Autodesk Inventor part; units mm, degrees
(part 9 of 11)
  line L1735 (12.5917, 6.0093) -> (11.97, 5.7878)
  arc A3472 (11.9573, 5.8237) -> (11.9828, 5.7519) centre (11.97, 5.7878) ccw
  arc A3473 (12.6045, 5.9734) -> (12.579, 6.0452) centre (12.5917, 6.0093) ccw
  line L1736 (11.97, 5.7878) -> (11.3254, 5.6466)
  arc A3474 (11.3172, 5.6838) -> (11.3335, 5.6094) centre (11.3254, 5.6466) ccw
  arc A3475 (11.9782, 5.7506) -> (11.9619, 5.825) centre (11.97, 5.7878) ccw
  line L1737 (11.3254, 5.6466) -> (10.668, 5.588)
  arc A3476 (10.6646, 5.626) -> (10.6714, 5.5501) centre (10.668, 5.588) ccw
  arc A3477 (11.3288, 5.6087) -> (11.322, 5.6846) centre (11.3254, 5.6466) ccw
  line L1738 (10.668, 5.588) -> (10.668, 6.858)
  arc A3478 (10.7061, 6.858) -> (10.6299, 6.858) centre (10.668, 6.858) ccw
  arc A3479 (10.6299, 5.588) -> (10.7061, 5.588) centre (10.668, 5.588) ccw
  line L1739 (10.668, 6.858) -> (11.1934, 6.8774)
  arc A3480 (11.1948, 6.8393) -> (11.192, 6.9155) centre (11.1934, 6.8774) ccw
  arc A3481 (10.6666, 6.8961) -> (10.6694, 6.8199) centre (10.668, 6.858) ccw
  line L1740 (11.1934, 6.8774) -> (11.7108, 6.9714)
  arc A3482 (11.7176, 6.9339) -> (11.704, 7.0089) centre (11.7108, 6.9714) ccw
  arc A3483 (11.1866, 6.9149) -> (11.2003, 6.8399) centre (11.1934, 6.8774) ccw
  line L1741 (11.7108, 6.9714) -> (12.2094, 7.1381)
  arc A3484 (12.2215, 7.1019) -> (12.1974, 7.1742) centre (12.2094, 7.1381) ccw
  arc A3485 (11.6987, 7.0075) -> (11.7228, 6.9353) centre (11.7108, 6.9714) ccw
  line L1742 (12.2094, 7.1381) -> (12.6793, 7.374)
  arc A3486 (12.6964, 7.34) -> (12.6623, 7.4081) centre (12.6794, 7.374) ccw
  arc A3487 (12.1924, 7.1721) -> (12.2265, 7.104) centre (12.2094, 7.1381) ccw
  line L1743 (12.6793, 7.374) -> (13.1109, 7.6744)
  arc A3488 (13.1326, 7.6431) -> (13.0891, 7.7057) centre (13.1109, 7.6744) ccw
  arc A3489 (12.6576, 7.4053) -> (12.7011, 7.3427) centre (12.6793, 7.374) ccw
  line L1744 (13.1109, 7.6744) -> (13.4952, 8.0332)
  arc A3490 (13.5212, 8.0053) -> (13.4693, 8.061) centre (13.4952, 8.0332) ccw
  arc A3491 (13.0849, 7.7023) -> (13.1369, 7.6465) centre (13.1109, 7.6744) ccw
  line L1745 (13.4952, 8.0332) -> (13.8247, 8.443)
  arc A3492 (13.8544, 8.4191) -> (13.795, 8.4669) centre (13.8247, 8.443) ccw
  arc A3493 (13.4655, 8.057) -> (13.5249, 8.0093) centre (13.4952, 8.0332) ccw
  line L1746 (13.8247, 8.443) -> (14.0924, 8.8955)
  arc A3494 (14.1252, 8.8761) -> (14.0596, 8.9149) centre (14.0924, 8.8955) ccw
  arc A3495 (13.7919, 8.4624) -> (13.8575, 8.4236) centre (13.8247, 8.443) ccw
  line L1747 (14.0924, 8.8955) -> (14.293, 9.3815)
  arc A3496 (14.3282, 9.367) -> (14.2578, 9.3961) centre (14.293, 9.3815) ccw
  arc A3497 (14.0572, 8.91) -> (14.1276, 8.881) centre (14.0924, 8.8955) ccw
  line L1748 (14.293, 9.3815) -> (14.4224, 9.8911)
  arc A3498 (14.4594, 9.8818) -> (14.3855, 9.9005) centre (14.4224, 9.8911) ccw
  arc A3499 (14.2561, 9.3909) -> (14.33, 9.3721) centre (14.293, 9.3815) ccw
  line L1749 (14.4224, 9.8911) -> (14.478, 10.414)
  arc A3500 (14.5159, 10.41) -> (14.4401, 10.418) centre (14.478, 10.414) ccw
  arc A3501 (14.3845, 9.8952) -> (14.4603, 9.8871) centre (14.4224, 9.8911) ccw
  line L1750 (14.478, 10.414) -> (14.478, 10.668)
  arc A3502 (14.5161, 10.668) -> (14.4399, 10.668) centre (14.478, 10.668) ccw
  arc A3503 (14.4399, 10.414) -> (14.5161, 10.414) centre (14.478, 10.414) ccw
  line L1751 (14.478, 10.668) -> (14.4392, 11.2102)
  arc A3504 (14.4772, 11.2129) -> (14.4012, 11.2075) centre (14.4392, 11.2102) ccw
  arc A3505 (14.44, 10.6653) -> (14.516, 10.6707) centre (14.478, 10.668) ccw
  line L1752 (14.4392, 11.2102) -> (14.3237, 11.7414)
  arc A3506 (14.3609, 11.7495) -> (14.2864, 11.7333) centre (14.3237, 11.7414) ccw
  arc A3507 (14.402, 11.2021) -> (14.4764, 11.2183) centre (14.4392, 11.2102) ccw
  line L1753 (14.3237, 11.7414) -> (14.1337, 12.2507)
  arc A3508 (14.1694, 12.264) -> (14.098, 12.2374) centre (14.1337, 12.2507) ccw
  arc A3509 (14.288, 11.7281) -> (14.3594, 11.7547) centre (14.3237, 11.7414) ccw
  line L1754 (14.1337, 12.2507) -> (13.8732, 12.7278)
  arc A3510 (13.9066, 12.7461) -> (13.8397, 12.7096) centre (13.8732, 12.7278) ccw
  arc A3511 (14.1003, 12.2325) -> (14.1671, 12.269) centre (14.1337, 12.2507) ccw
  line L1755 (13.8732, 12.7278) -> (13.5474, 13.163)
  arc A3512 (13.5779, 13.1859) -> (13.5169, 13.1402) centre (13.5474, 13.163) ccw
  arc A3513 (13.8427, 12.705) -> (13.9037, 12.7507) centre (13.8732, 12.7278) ccw
  line L1756 (13.5474, 13.163) -> (13.163, 13.5474)
  arc A3514 (13.19, 13.5743) -> (13.1361, 13.5205) centre (13.163, 13.5474) ccw
  arc A3515 (13.5205, 13.1361) -> (13.5743, 13.19) centre (13.5474, 13.163) ccw
  line L1757 (13.163, 13.5474) -> (12.7278, 13.8732)
  arc A3516 (12.7507, 13.9037) -> (12.705, 13.8427) centre (12.7278, 13.8732) ccw
  arc A3517 (13.1402, 13.5169) -> (13.1859, 13.5779) centre (13.163, 13.5474) ccw
  line L1758 (12.7278, 13.8732) -> (12.2507, 14.1337)
  arc A3518 (12.269, 14.1671) -> (12.2325, 14.1003) centre (12.2507, 14.1337) ccw
  arc A3519 (12.7096, 13.8397) -> (12.7461, 13.9066) centre (12.7278, 13.8732) ccw
  line L1759 (12.2507, 14.1337) -> (11.7414, 14.3237)
  arc A3520 (11.7547, 14.3594) -> (11.7281, 14.288) centre (11.7414, 14.3237) ccw
  arc A3521 (12.2374, 14.098) -> (12.264, 14.1694) centre (12.2507, 14.1337) ccw
  line L1760 (11.7414, 14.3237) -> (11.2102, 14.4392)
  arc A3522 (11.2183, 14.4764) -> (11.2021, 14.402) centre (11.2102, 14.4392) ccw
  arc A3523 (11.7333, 14.2864) -> (11.7495, 14.3609) centre (11.7414, 14.3237) ccw
  line L1761 (11.2102, 14.4392) -> (10.668, 14.478)
  arc A3524 (10.6707, 14.516) -> (10.6653, 14.44) centre (10.668, 14.478) ccw
  arc A3525 (11.2075, 14.4012) -> (11.2129, 14.4772) centre (11.2102, 14.4392) ccw
  line L1762 (10.668, 14.478) -> (10.1258, 14.4392)
  arc A3526 (10.1231, 14.4772) -> (10.1285, 14.4012) centre (10.1258, 14.4392) ccw
  arc A3527 (10.6707, 14.44) -> (10.6653, 14.516) centre (10.668, 14.478) ccw
  line L1763 (10.1258, 14.4392) -> (9.5946, 14.3237)
  arc A3528 (9.5865, 14.3609) -> (9.6027, 14.2864) centre (9.5946, 14.3237) ccw
  arc A3529 (10.1339, 14.402) -> (10.1177, 14.4764) centre (10.1258, 14.4392) ccw
  line L1764 (9.5946, 14.3237) -> (9.0853, 14.1337)
  arc A3530 (9.072, 14.1694) -> (9.0986, 14.098) centre (9.0853, 14.1337) ccw
  arc A3531 (9.6079, 14.288) -> (9.5813, 14.3593) centre (9.5946, 14.3237) ccw
  line L1765 (9.0853, 14.1337) -> (8.6082, 13.8732)
  arc A3532 (8.5899, 13.9066) -> (8.6264, 13.8397) centre (8.6082, 13.8732) ccw
  arc A3533 (9.1035, 14.1003) -> (9.067, 14.1671) centre (9.0853, 14.1337) ccw
  line L1766 (8.6082, 13.8732) -> (8.173, 13.5474)
  arc A3534 (8.1501, 13.5779) -> (8.1958, 13.5169) centre (8.173, 13.5474) ccw
  arc A3535 (8.631, 13.8427) -> (8.5853, 13.9037) centre (8.6082, 13.8732) ccw
  line L1767 (8.173, 13.5474) -> (7.7886, 13.163)
  arc A3536 (7.7617, 13.19) -> (7.8155, 13.1361) centre (7.7886, 13.163) ccw
  arc A3537 (8.1999, 13.5205) -> (8.146, 13.5743) centre (8.173, 13.5474) ccw
  line L1768 (7.7886, 13.163) -> (7.4628, 12.7278)
  arc A3538 (7.4323, 12.7507) -> (7.4933, 12.705) centre (7.4628, 12.7278) ccw
  arc A3539 (7.8191, 13.1402) -> (7.7581, 13.1859) centre (7.7886, 13.163) ccw
  line L1769 (7.4628, 12.7278) -> (7.2023, 12.2507)
  arc A3540 (7.1689, 12.269) -> (7.2357, 12.2325) centre (7.2023, 12.2507) ccw
  arc A3541 (7.4963, 12.7096) -> (7.4294, 12.7461) centre (7.4628, 12.7278) ccw
  line L1770 (7.2023, 12.2507) -> (7.0123, 11.7414)
  arc A3542 (6.9766, 11.7547) -> (7.048, 11.7281) centre (7.0123, 11.7414) ccw
  arc A3543 (7.238, 12.2374) -> (7.1666, 12.264) centre (7.2023, 12.2507) ccw
  line L1771 (7.0123, 11.7414) -> (6.8968, 11.2102)
  arc A3544 (6.8596, 11.2183) -> (6.934, 11.2021) centre (6.8968, 11.2102) ccw
  arc A3545 (7.0496, 11.7333) -> (6.9751, 11.7495) centre (7.0123, 11.7414) ccw
  line L1772 (6.8968, 11.2102) -> (6.858, 10.668)
  arc A3546 (6.82, 10.6707) -> (6.896, 10.6653) centre (6.858, 10.668) ccw
  arc A3547 (6.9348, 11.2075) -> (6.8588, 11.2129) centre (6.8968, 11.2102) ccw
  line L1773 (6.858, 10.668) -> (6.8782, 10.1815)
  arc A3548 (6.8402, 10.18) -> (6.9163, 10.1831) centre (6.8782, 10.1815) ccw
  arc A3549 (6.8961, 10.6696) -> (6.8199, 10.6664) centre (6.858, 10.668) ccw
  line L1774 (6.8782, 10.1815) -> (6.9618, 9.7019)
  arc A3550 (6.9242, 9.6953) -> (6.9993, 9.7084) centre (6.9618, 9.7019) ccw
  arc A3551 (6.9158, 10.1881) -> (6.8407, 10.175) centre (6.8782, 10.1815) ccw
  line L1775 (6.9618, 9.7019) -> (7.1072, 9.2372)
  arc A3552 (7.0709, 9.2258) -> (7.1436, 9.2486) centre (7.1072, 9.2372) ccw
  arc A3553 (6.9982, 9.7133) -> (6.9254, 9.6905) centre (6.9618, 9.7019) ccw
  line L1776 (7.1072, 9.2372) -> (7.3121, 8.7955)
  arc A3554 (7.2775, 8.7795) -> (7.3466, 8.8116) centre (7.3121, 8.7955) ccw
  arc A3555 (7.1418, 9.2533) -> (7.0727, 9.2212) centre (7.1072, 9.2372) ccw
  line L1777 (7.3121, 8.7955) -> (7.5728, 8.3843)
  arc A3556 (7.5407, 8.364) -> (7.605, 8.4047) centre (7.5728, 8.3843) ccw
  arc A3557 (7.3443, 8.8159) -> (7.2799, 8.7751) centre (7.3121, 8.7955) ccw
  line L1778 (7.5728, 8.3843) -> (7.885, 8.0107)
  arc A3558 (7.8558, 7.9863) -> (7.9143, 8.0352) centre (7.885, 8.0107) ccw
  arc A3559 (7.6021, 8.4088) -> (7.5436, 8.3599) centre (7.5728, 8.3843) ccw
  line L1779 (7.885, 8.0107) -> (8.2433, 7.6811)
  arc A3560 (8.2175, 7.653) -> (8.2691, 7.7091) centre (8.2433, 7.6811) ccw
  arc A3561 (7.9108, 8.0388) -> (7.8592, 7.9827) centre (7.885, 8.0107) ccw
  line L1780 (8.2433, 7.6811) -> (8.6416, 7.401)
  arc A3562 (8.6196, 7.3698) -> (8.6635, 7.4321) centre (8.6416, 7.401) ccw
  arc A3563 (8.2652, 7.7122) -> (8.2214, 7.6499) centre (8.2433, 7.6811) ccw
  line L1781 (8.6416, 7.401) -> (9.073, 7.1753)
  arc A3564 (9.0553, 7.1415) -> (9.0906, 7.209) centre (9.073, 7.1753) ccw
  arc A3565 (8.6592, 7.4347) -> (8.6239, 7.3672) centre (8.6416, 7.401) ccw
  line L1782 (9.073, 7.1753) -> (9.27, 7.6205)
  arc A3566 (9.517, 6.972) -> (9.5432, 7.0436) centre (9.5301, 7.0078) ccw
  arc A3567 (9.0861, 7.211) -> (9.0599, 7.1395) centre (9.073, 7.1753) ccw
  line L1783 (9.27, 7.6205) -> (9.4072, 8.0877)
  arc A3568 (9.3988, 8.0505) -> (9.4155, 8.1249) centre (9.4072, 8.0877) ccw
  arc A3569 (9.2783, 7.6577) -> (9.2616, 7.5833) centre (9.27, 7.6205) ccw
  line L1784 (9.4072, 8.0877) -> (10.4902, 6.858)
  arc A3570 (10.4868, 6.8201) -> (10.4936, 6.896) centre (10.4902, 6.858) ccw
  arc A3571 (9.4106, 8.1256) -> (9.4038, 8.0497) centre (9.4072, 8.0877) ccw
  line L1785 (10.4902, 6.858) -> (10.4902, 5.588)
  arc A3572 (10.4521, 5.588) -> (10.5283, 5.588) centre (10.4902, 5.588) ccw
  arc A3573 (10.5283, 6.858) -> (10.4521, 6.858) centre (10.4902, 6.858) ccw
  line L1786 (9.9806, 15.6972) -> (11.3554, 15.6972)
  arc A3574 (11.3554, 15.6591) -> (11.3554, 15.7353) centre (11.3554, 15.6972) ccw
  arc A3575 (9.9806, 15.7353) -> (9.9806, 15.6591) centre (9.9806, 15.6972) ccw
  line L1787 (9.2739, 15.5448) -> (12.0621, 15.5448)
  arc A3576 (12.0621, 15.5067) -> (12.0621, 15.5829) centre (12.0621, 15.5448) ccw
  arc A3577 (9.2739, 15.5829) -> (9.2739, 15.5067) centre (9.2739, 15.5448) ccw
  line L1788 (8.81, 15.3924) -> (12.526, 15.3924)
  arc A3578 (12.526, 15.3543) -> (12.526, 15.4305) centre (12.526, 15.3924) ccw
  arc A3579 (8.81, 15.4305) -> (8.81, 15.3543) centre (8.81, 15.3924) ccw
  line L1789 (8.4714, 15.24) -> (12.8646, 15.24)
  arc A3580 (12.8646, 15.2019) -> (12.8646, 15.2781) centre (12.8646, 15.24) ccw
  arc A3581 (8.4714, 15.2781) -> (8.4714, 15.2019) centre (8.4714, 15.24) ccw
  line L1790 (8.1773, 15.0876) -> (13.1587, 15.0876)
  arc A3582 (13.1587, 15.0495) -> (13.1587, 15.1257) centre (13.1587, 15.0876) ccw
  arc A3583 (8.1773, 15.1257) -> (8.1773, 15.0495) centre (8.1773, 15.0876) ccw
  line L1791 (7.9252, 14.9352) -> (13.4108, 14.9352)
  arc A3584 (13.4108, 14.8971) -> (13.4108, 14.9733) centre (13.4108, 14.9352) ccw
  arc A3585 (7.9252, 14.9733) -> (7.9252, 14.8971) centre (7.9252, 14.9352) ccw
  line L1792 (7.698, 14.7828) -> (13.638, 14.7828)
  arc A3586 (13.638, 14.7447) -> (13.638, 14.8209) centre (13.638, 14.7828) ccw
  arc A3587 (7.698, 14.8209) -> (7.698, 14.7447) centre (7.698, 14.7828) ccw
  line L1793 (7.5035, 14.6304) -> (13.8325, 14.6304)
  arc A3588 (13.8325, 14.5923) -> (13.8325, 14.6685) centre (13.8325, 14.6304) ccw
  arc A3589 (7.5035, 14.6685) -> (7.5035, 14.5923) centre (7.5035, 14.6304) ccw
  line L1794 (7.309, 14.478) -> (10.668, 14.478)
  arc A3590 (10.668, 14.4399) -> (10.668, 14.5161) centre (10.668, 14.478) ccw
  arc A3591 (7.309, 14.5161) -> (7.309, 14.4399) centre (7.309, 14.478) ccw
  line L1795 (10.668, 14.478) -> (14.027, 14.478)
  arc A3592 (14.027, 14.4399) -> (14.027, 14.5161) centre (14.027, 14.478) ccw
  arc A3593 (10.668, 14.5161) -> (10.668, 14.4399) centre (10.668, 14.478) ccw
  line L1796 (7.1545, 14.3256) -> (9.6035, 14.3256)
  arc A3594 (9.6035, 14.2875) -> (9.6035, 14.3637) centre (9.6035, 14.3256) ccw
  arc A3595 (7.1545, 14.3637) -> (7.1545, 14.2875) centre (7.1545, 14.3256) ccw
  line L1797 (11.7325, 14.3256) -> (14.1815, 14.3256)
  arc A3596 (14.1815, 14.2875) -> (14.1815, 14.3637) centre (14.1815, 14.3256) ccw
  arc A3597 (11.7325, 14.3637) -> (11.7325, 14.2875) centre (11.7325, 14.3256) ccw
  line L1798 (7.0021, 14.1732) -> (9.1912, 14.1732)
  arc A3598 (9.1912, 14.1351) -> (9.1912, 14.2113) centre (9.1912, 14.1732) ccw
  arc A3599 (7.0021, 14.2113) -> (7.0021, 14.1351) centre (7.0021, 14.1732) ccw
  line L1799 (12.1448, 14.1732) -> (14.3339, 14.1732)
  arc A3600 (14.3339, 14.1351) -> (14.3339, 14.2113) centre (14.3339, 14.1732) ccw
  arc A3601 (12.1448, 14.2113) -> (12.1448, 14.1351) centre (12.1448, 14.1732) ccw
  line L1800 (6.8532, 14.0208) -> (8.8785, 14.0208)
  arc A3602 (8.8785, 13.9827) -> (8.8785, 14.0589) centre (8.8785, 14.0208) ccw
  arc A3603 (6.8532, 14.0589) -> (6.8532, 13.9827) centre (6.8532, 14.0208) ccw
  line L1801 (12.4575, 14.0208) -> (14.4829, 14.0208)
  arc A3604 (14.4829, 13.9827) -> (14.4829, 14.0589) centre (14.4829, 14.0208) ccw
  arc A3605 (12.4575, 14.0589) -> (12.4575, 13.9827) centre (12.4575, 14.0208) ccw
  line L1802 (6.7337, 13.8684) -> (8.6018, 13.8684)
  arc A3606 (8.6018, 13.8303) -> (8.6018, 13.9065) centre (8.6018, 13.8684) ccw
  arc A3607 (6.7337, 13.9065) -> (6.7337, 13.8303) centre (6.7337, 13.8684) ccw
  line L1803 (12.7342, 13.8684) -> (14.6023, 13.8684)
  arc A3608 (14.6023, 13.8303) -> (14.6023, 13.9065) centre (14.6023, 13.8684) ccw
  arc A3609 (12.7342, 13.9065) -> (12.7342, 13.8303) centre (12.7342, 13.8684) ccw
  line L1804 (6.6143, 13.716) -> (8.3982, 13.716)
  arc A3610 (8.3982, 13.6779) -> (8.3982, 13.7541) centre (8.3982, 13.716) ccw
  arc A3611 (6.6143, 13.7541) -> (6.6143, 13.6779) centre (6.6143, 13.716) ccw
  line L1805 (12.9378, 13.716) -> (14.7217, 13.716)
  arc A3612 (14.7217, 13.6779) -> (14.7217, 13.7541) centre (14.7217, 13.716) ccw
  arc A3613 (12.9378, 13.7541) -> (12.9378, 13.6779) centre (12.9378, 13.716) ccw
  line L1806 (6.4949, 13.5636) -> (8.1946, 13.5636)
  arc A3614 (8.1946, 13.5255) -> (8.1946, 13.6017) centre (8.1946, 13.5636) ccw
  arc A3615 (6.4949, 13.6017) -> (6.4949, 13.5255) centre (6.4949, 13.5636) ccw
  line L1807 (13.1414, 13.5636) -> (14.8411, 13.5636)
  arc A3616 (14.8411, 13.5255) -> (14.8411, 13.6017) centre (14.8411, 13.5636) ccw
  arc A3617 (13.1414, 13.6017) -> (13.1414, 13.5255) centre (13.1414, 13.5636) ccw
  line L1808 (6.4011, 13.4112) -> (8.0368, 13.4112)
  arc A3618 (8.0368, 13.3731) -> (8.0368, 13.4493) centre (8.0368, 13.4112) ccw
  arc A3619 (6.4011, 13.4493) -> (6.4011, 13.3731) centre (6.4011, 13.4112) ccw
  line L1809 (13.2992, 13.4113) -> (14.935, 13.4112)
  arc A3620 (14.935, 13.3731) -> (14.935, 13.4493) centre (14.935, 13.4112) ccw
  arc A3621 (13.2992, 13.4494) -> (13.2992, 13.3732) centre (13.2992, 13.4113) ccw
  line L1810 (6.3089, 13.2588) -> (7.8844, 13.2588)
  arc A3622 (7.8844, 13.2207) -> (7.8844, 13.2969) centre (7.8844, 13.2588) ccw
  arc A3623 (6.3089, 13.2969) -> (6.3089, 13.2207) centre (6.3089, 13.2588) ccw
  line L1811 (13.4516, 13.2589) -> (15.0271, 13.2588)
  arc A3624 (15.0271, 13.2207) -> (15.0271, 13.2969) centre (15.0271, 13.2588) ccw
  arc A3625 (13.4516, 13.297) -> (13.4516, 13.2208) centre (13.4516, 13.2589) ccw
  line L1812 (6.2168, 13.1064) -> (7.7463, 13.1064)
  arc A3626 (7.7463, 13.0683) -> (7.7463, 13.1445) centre (7.7463, 13.1064) ccw
  arc A3627 (6.2168, 13.1445) -> (6.2168, 13.0683) centre (6.2168, 13.1064) ccw
  line L1813 (13.5898, 13.1064) -> (15.1192, 13.1064)
  arc A3628 (15.1192, 13.0683) -> (15.1192, 13.1445) centre (15.1192, 13.1064) ccw
  arc A3629 (13.5898, 13.1445) -> (13.5898, 13.0683) centre (13.5898, 13.1064) ccw
  line L1814 (6.1362, 12.954) -> (7.6321, 12.954)
  arc A3630 (7.6321, 12.9159) -> (7.6321, 12.9921) centre (7.6321, 12.954) ccw
  arc A3631 (6.1362, 12.9921) -> (6.1362, 12.9159) centre (6.1362, 12.954) ccw
  line L1815 (13.7039, 12.9541) -> (15.1998, 12.954)
  arc A3632 (15.1998, 12.9159) -> (15.1998, 12.9921) centre (15.1998, 12.954) ccw
  arc A3633 (13.7039, 12.9922) -> (13.7039, 12.916) centre (13.7039, 12.9541) ccw
  line L1816 (6.0676, 12.8016) -> (7.5181, 12.8016)
  arc A3634 (7.5181, 12.7635) -> (7.5181, 12.8397) centre (7.5181, 12.8016) ccw
  arc A3635 (6.0676, 12.8397) -> (6.0676, 12.7635) centre (6.0676, 12.8016) ccw
  line L1817 (13.818, 12.8016) -> (15.2683, 12.8016)
  arc A3636 (15.2683, 12.7635) -> (15.2683, 12.8397) centre (15.2683, 12.8016) ccw
  arc A3637 (13.818, 12.8397) -> (13.818, 12.7635) centre (13.818, 12.8016) ccw
  line L1818 (5.9991, 12.6492) -> (7.4199, 12.6492)
  arc A3638 (7.4199, 12.6111) -> (7.4199, 12.6873) centre (7.4199, 12.6492) ccw
  arc A3639 (5.9991, 12.6873) -> (5.9991, 12.6111) centre (5.9991, 12.6492) ccw
  line L1819 (13.9161, 12.6492) -> (15.3369, 12.6492)
  arc A3640 (15.3369, 12.6111) -> (15.3369, 12.6873) centre (15.3369, 12.6492) ccw
  arc A3641 (13.9161, 12.6873) -> (13.9161, 12.6111) centre (13.9161, 12.6492) ccw
  line L1820 (5.9305, 12.4968) -> (7.3367, 12.4968)
  arc A3642 (7.3367, 12.4587) -> (7.3367, 12.5349) centre (7.3367, 12.4968) ccw
  arc A3643 (5.9305, 12.5349) -> (5.9305, 12.4587) centre (5.9305, 12.4968) ccw
  line L1821 (13.9993, 12.4968) -> (15.4055, 12.4968)
  arc A3644 (15.4055, 12.4587) -> (15.4055, 12.5349) centre (15.4055, 12.4968) ccw
  arc A3645 (13.9993, 12.5349) -> (13.9993, 12.4587) centre (13.9993, 12.4968) ccw
  line L1822 (5.8792, 12.3444) -> (7.2535, 12.3444)
  arc A3646 (7.2535, 12.3063) -> (7.2535, 12.3825) centre (7.2535, 12.3444) ccw
  arc A3647 (5.8792, 12.3825) -> (5.8792, 12.3063) centre (5.8792, 12.3444) ccw
  line L1823 (14.0825, 12.3444) -> (15.4568, 12.3444)
  arc A3648 (15.4568, 12.3063) -> (15.4568, 12.3825) centre (15.4568, 12.3444) ccw
  arc A3649 (14.0825, 12.3825) -> (14.0825, 12.3063) centre (14.0825, 12.3444) ccw
  line L1824 (5.8317, 12.192) -> (7.1804, 12.192)
  arc A3650 (7.1804, 12.1539) -> (7.1804, 12.2301) centre (7.1804, 12.192) ccw
  arc A3651 (5.8317, 12.2301) -> (5.8317, 12.1539) centre (5.8317, 12.192) ccw
  line L1825 (14.1556, 12.192) -> (15.5043, 12.192)
  arc A3652 (15.5043, 12.1539) -> (15.5043, 12.2301) centre (15.5043, 12.192) ccw
  arc A3653 (14.1556, 12.2301) -> (14.1556, 12.1539) centre (14.1556, 12.192) ccw
  line L1826 (5.7842, 12.0396) -> (7.1236, 12.0396)
  arc A3654 (7.1236, 12.0015) -> (7.1236, 12.0777) centre (7.1236, 12.0396) ccw
  arc A3655 (5.7842, 12.0777) -> (5.7842, 12.0015) centre (5.7842, 12.0396) ccw
  line L1827 (14.2124, 12.0396) -> (15.5518, 12.0396)
  arc A3656 (15.5518, 12.0015) -> (15.5518, 12.0777) centre (15.5518, 12.0396) ccw
  arc A3657 (14.2124, 12.0777) -> (14.2124, 12.0015) centre (14.2124, 12.0396) ccw
  line L1828 (5.7367, 11.8872) -> (7.0667, 11.8872)
  arc A3658 (7.0667, 11.8491) -> (7.0667, 11.9253) centre (7.0667, 11.8872) ccw
  arc A3659 (5.7367, 11.9253) -> (5.7367, 11.8491) centre (5.7367, 11.8872) ccw
  line L1829 (14.2693, 11.8872) -> (15.5993, 11.8872)
  arc A3660 (15.5993, 11.8491) -> (15.5993, 11.9253) centre (15.5993, 11.8872) ccw
  arc A3661 (14.2693, 11.9253) -> (14.2693, 11.8491) centre (14.2693, 11.8872) ccw
  line L1830 (5.7083, 11.7348) -> (7.0109, 11.7348)
  arc A3662 (7.0109, 11.6967) -> (7.0109, 11.7729) centre (7.0109, 11.7348) ccw
  arc A3663 (5.7083, 11.7729) -> (5.7083, 11.6967) centre (5.7083, 11.7348) ccw
  line L1831 (14.3251, 11.7348) -> (15.6277, 11.7348)
  arc A3664 (15.6277, 11.6967) -> (15.6277, 11.7729) centre (15.6277, 11.7348) ccw
  arc A3665 (14.3251, 11.7729) -> (14.3251, 11.6967) centre (14.3251, 11.7348) ccw
  line L1832 (5.6804, 11.5824) -> (6.9777, 11.5824)
  arc A3666 (6.9777, 11.5443) -> (6.9777, 11.6205) centre (6.9777, 11.5824) ccw
  arc A3667 (5.6804, 11.6205) -> (5.6804, 11.5443) centre (5.6804, 11.5824) ccw
  line L1833 (14.3583, 11.5824) -> (15.6557, 11.5824)
  arc A3668 (15.6557, 11.5443) -> (15.6557, 11.6205) centre (15.6557, 11.5824) ccw
  arc A3669 (14.3583, 11.6205) -> (14.3583, 11.5443) centre (14.3583, 11.5824) ccw
  line L1834 (5.6525, 11.43) -> (6.9446, 11.43)
  arc A3670 (6.9446, 11.3919) -> (6.9446, 11.4681) centre (6.9446, 11.43) ccw
  arc A3671 (5.6525, 11.4681) -> (5.6525, 11.3919) centre (5.6525, 11.43) ccw
  line L1835 (14.3914, 11.43) -> (15.6837, 11.43)
  arc A3672 (15.6837, 11.3919) -> (15.6837, 11.4681) centre (15.6837, 11.43) ccw
  arc A3673 (14.3914, 11.4681) -> (14.3914, 11.3919) centre (14.3914, 11.43) ccw
  line L1836 (5.6249, 11.2776) -> (6.9114, 11.2776)
  arc A3674 (6.9114, 11.2395) -> (6.9114, 11.3157) centre (6.9114, 11.2776) ccw
  arc A3675 (5.6249, 11.3157) -> (5.6249, 11.2395) centre (5.6249, 11.2776) ccw
  line L1837 (14.4246, 11.2776) -> (15.7111, 11.2776)
  arc A3676 (15.7111, 11.2395) -> (15.7111, 11.3157) centre (15.7111, 11.2776) ccw
  arc A3677 (14.4246, 11.3157) -> (14.4246, 11.2395) centre (14.4246, 11.2776) ccw
  line L1838 (5.6157, 11.1252) -> (6.8907, 11.1252)
  arc A3678 (6.8907, 11.0871) -> (6.8907, 11.1633) centre (6.8907, 11.1252) ccw
  arc A3679 (5.6157, 11.1633) -> (5.6157, 11.0871) centre (5.6157, 11.1252) ccw
  line L1839 (14.4455, 11.1257) -> (15.7205, 11.1252)
  arc A3680 (15.7205, 11.0871) -> (15.7205, 11.1633) centre (15.7205, 11.1252) ccw
  arc A3681 (14.4455, 11.1638) -> (14.4455, 11.0876) centre (14.4455, 11.1257) ccw
  line L1840 (5.6064, 10.9728) -> (6.8798, 10.9728)
  arc A3682 (6.8798, 10.9347) -> (6.8798, 11.0109) centre (6.8798, 10.9728) ccw
  arc A3683 (5.6064, 11.0109) -> (5.6064, 10.9347) centre (5.6064, 10.9728) ccw
  line L1841 (14.4562, 10.9728) -> (15.7297, 10.9728)
  arc A3684 (15.7297, 10.9347) -> (15.7297, 11.0109) centre (15.7297, 10.9728) ccw
  arc A3685 (14.4562, 11.0109) -> (14.4562, 10.9347) centre (14.4562, 10.9728) ccw
  line L1842 (5.5972, 10.8204) -> (6.8689, 10.8204)
  arc A3686 (6.8689, 10.7823) -> (6.8689, 10.8585) centre (6.8689, 10.8204) ccw
  arc A3687 (5.5972, 10.8585) -> (5.5972, 10.7823) centre (5.5972, 10.8204) ccw
  line L1843 (14.4671, 10.8204) -> (15.7388, 10.8204)
  arc A3688 (15.7388, 10.7823) -> (15.7388, 10.8585) centre (15.7388, 10.8204) ccw
  arc A3689 (14.4671, 10.8585) -> (14.4671, 10.7823) centre (14.4671, 10.8204) ccw
  line L1844 (5.588, 10.668) -> (6.858, 10.668)
  arc A3690 (6.858, 10.6299) -> (6.858, 10.7061) centre (6.858, 10.668) ccw
  arc A3691 (5.588, 10.7061) -> (5.588, 10.6299) centre (5.588, 10.668) ccw
  line L1845 (14.478, 10.668) -> (15.748, 10.668)
  arc A3692 (15.748, 10.6299) -> (15.748, 10.7061) centre (15.748, 10.668) ccw
  arc A3693 (14.478, 10.7061) -> (14.478, 10.6299) centre (14.478, 10.668) ccw
  line L1846 (5.5953, 10.5156) -> (6.8643, 10.5156)
  arc A3694 (6.8643, 10.4775) -> (6.8643, 10.5537) centre (6.8643, 10.5156) ccw
  arc A3695 (5.5953, 10.5537) -> (5.5953, 10.4775) centre (5.5953, 10.5156) ccw
  line L1847 (14.478, 10.5156) -> (15.7344, 10.5156)
  arc A3696 (15.7344, 10.4775) -> (15.7344, 10.5537) centre (15.7344, 10.5156) ccw
  arc A3697 (14.478, 10.5537) -> (14.478, 10.4775) centre (14.478, 10.5156) ccw
  line L1848 (5.6025, 10.3632) -> (6.8707, 10.3632)
  arc A3698 (6.8707, 10.3251) -> (6.8707, 10.4013) centre (6.8707, 10.3632) ccw
  arc A3699 (5.6025, 10.4013) -> (5.6025, 10.3251) centre (5.6025, 10.3632) ccw
  line L1849 (14.4726, 10.3632) -> (15.7208, 10.3632)
  arc A3700 (15.7208, 10.3251) -> (15.7208, 10.4013) centre (15.7208, 10.3632) ccw
  arc A3701 (14.4726, 10.4013) -> (14.4726, 10.3251) centre (14.4726, 10.3632) ccw
  line L1850 (5.6098, 10.2108) -> (6.877, 10.2108)
  arc A3702 (6.877, 10.1727) -> (6.877, 10.2489) centre (6.877, 10.2108) ccw
  arc A3703 (5.6098, 10.2489) -> (5.6098, 10.1727) centre (5.6098, 10.2108) ccw
  line L1851 (14.4564, 10.2108) -> (15.7072, 10.2108)
  arc A3704 (15.7072, 10.1727) -> (15.7072, 10.2489) centre (15.7072, 10.2108) ccw
  arc A3705 (14.4564, 10.2489) -> (14.4564, 10.1727) centre (14.4564, 10.2108) ccw
  line L1852 (5.6171, 10.0584) -> (6.8997, 10.0584)
  arc A3706 (6.8997, 10.0203) -> (6.8997, 10.0965) centre (6.8997, 10.0584) ccw
  arc A3707 (5.6171, 10.0965) -> (5.6171, 10.0203) centre (5.6171, 10.0584) ccw
  line L1853 (14.4402, 10.0584) -> (15.6936, 10.0584)
  arc A3708 (15.6936, 10.0203) -> (15.6936, 10.0965) centre (15.6936, 10.0584) ccw
  arc A3709 (14.4402, 10.0965) -> (14.4402, 10.0203) centre (14.4402, 10.0584) ccw
  line L1854 (5.6389, 9.906) -> (6.9262, 9.906)
  arc A3710 (6.9262, 9.8679) -> (6.9262, 9.9441) centre (6.9262, 9.906) ccw
  arc A3711 (5.6389, 9.9441) -> (5.6389, 9.8679) centre (5.6389, 9.906) ccw
  line L1855 (14.424, 9.906) -> (15.6665, 9.906)
  arc A3712 (15.6665, 9.8679) -> (15.6665, 9.9441) centre (15.6665, 9.906) ccw
  arc A3713 (14.424, 9.9441) -> (14.424, 9.8679) centre (14.424, 9.906) ccw
  line L1856 (5.6664, 9.7536) -> (6.9528, 9.7536)
  arc A3714 (6.9528, 9.7155) -> (6.9528, 9.7917) centre (6.9528, 9.7536) ccw
  arc A3715 (5.6664, 9.7917) -> (5.6664, 9.7155) centre (5.6664, 9.7536) ccw
  line L1857 (14.3875, 9.7536) -> (15.6331, 9.7536)
  arc A3716 (15.6331, 9.7155) -> (15.6331, 9.7917) centre (15.6331, 9.7536) ccw
  arc A3717 (14.3875, 9.7917) -> (14.3875, 9.7155) centre (14.3875, 9.7536) ccw
  line L1858 (5.6939, 9.6012) -> (6.9933, 9.6012)
  arc A3718 (6.9933, 9.5631) -> (6.9933, 9.6393) centre (6.9933, 9.6012) ccw
  arc A3719 (5.6939, 9.6393) -> (5.6939, 9.5631) centre (5.6939, 9.6012) ccw
  line L1859 (14.3488, 9.6012) -> (15.5997, 9.6012)
  arc A3720 (15.5997, 9.5631) -> (15.5997, 9.6393) centre (15.5997, 9.6012) ccw
  arc A3721 (14.3488, 9.6393) -> (14.3488, 9.5631) centre (14.3488, 9.6012) ccw
  line L1860 (5.7214, 9.4488) -> (7.041, 9.4488)
  arc A3722 (7.041, 9.4107) -> (7.041, 9.4869) centre (7.041, 9.4488) ccw
  arc A3723 (5.7214, 9.4869) -> (5.7214, 9.4107) centre (5.7214, 9.4488) ccw
  line L1861 (14.3101, 9.4488) -> (15.5663, 9.4488)
  arc A3724 (15.5663, 9.4107) -> (15.5663, 9.4869) centre (15.5663, 9.4488) ccw
  arc A3725 (14.3101, 9.4869) -> (14.3101, 9.4107) centre (14.3101, 9.4488) ccw
  line L1862 (5.7596, 9.2964) -> (7.0887, 9.2964)
  arc A3726 (7.0887, 9.2583) -> (7.0887, 9.3345) centre (7.0887, 9.2964) ccw
  arc A3727 (5.7596, 9.3345) -> (5.7596, 9.2583) centre (5.7596, 9.2964) ccw
  line L1863 (14.2579, 9.2964) -> (15.5234, 9.2964)
  arc A3728 (15.5234, 9.2583) -> (15.5234, 9.3345) centre (15.5234, 9.2964) ccw
  arc A3729 (14.2579, 9.3345) -> (14.2579, 9.2583) centre (14.2579, 9.2964) ccw
  line L1864 (5.8083, 9.144) -> (7.1505, 9.144)
  arc A3730 (7.1505, 9.1059) -> (7.1505, 9.1821) centre (7.1505, 9.144) ccw
  arc A3731 (5.8083, 9.1821) -> (5.8083, 9.1059) centre (5.8083, 9.144) ccw
  line L1865 (14.195, 9.144) -> (15.4691, 9.144)
  arc A3732 (15.4691, 9.1059) -> (15.4691, 9.1821) centre (15.4691, 9.144) ccw
  arc A3733 (14.195, 9.1821) -> (14.195, 9.1059) centre (14.195, 9.144) ccw
  line L1866 (5.8571, 8.9916) -> (7.2211, 8.9916)
  arc A3734 (7.2211, 8.9535) -> (7.2211, 9.0297) centre (7.2211, 8.9916) ccw
  arc A3735 (5.8571, 9.0297) -> (5.8571, 8.9535) centre (5.8571, 8.9916) ccw
  line L1867 (14.1321, 8.9916) -> (15.4149, 8.9916)
  arc A3736 (15.4149, 8.9535) -> (15.4149, 9.0297) centre (15.4149, 8.9916) ccw
  arc A3737 (14.1321, 9.0297) -> (14.1321, 8.9535) centre (14.1321, 8.9916) ccw
  line L1868 (5.9058, 8.8392) -> (7.2918, 8.8392)
  arc A3738 (7.2918, 8.8011) -> (7.2918, 8.8773) centre (7.2918, 8.8392) ccw
  arc A3739 (5.9058, 8.8773) -> (5.9058, 8.8011) centre (5.9058, 8.8392) ccw
  line L1869 (14.0591, 8.8392) -> (15.3606, 8.8392)
  constraints: 8878 point on circle, 3740 centre point, 3708 end point, 1915 point on line, 448 other
sketch "20" plane through (0, 0, 0) normal (0, 0, 1) x (1, 0, 0)
  arc A0 (-0.1016, 13) -> (0.1016, 13) centre (0, 13) ccw
  arc A1 (0.1016, 31.75) -> (-0.1016, 31.75) centre (0, 31.75) ccw
  line L0 (0, 6.5) -> (0, 4.1271)
  arc A2 (-0.1016, 4.1271) -> (0.1016, 4.1271) centre (0, 4.1271) ccw
  arc A3 (0.1016, 6.5) -> (-0.1016, 6.5) centre (0, 6.5) ccw
  arc A4 (0, 4.1271) -> (5.1431, 0) centre (4.6351, 4.6351) ccw
  arc A5 (0.101, 4.1382) -> (-0.101, 4.116) centre (0, 4.1271) ccw
  arc A6 (5.1542, -0.101) -> (5.132, 0.101) centre (5.1431, 0) ccw
  line L1 (5.1431, 0) -> (6.5, 0)
  arc A7 (6.5, -0.1016) -> (6.5, 0.1016) centre (6.5, 0) ccw
  arc A8 (5.1431, 0.1016) -> (5.1431, -0.1016) centre (5.1431, 0) ccw
  line L2 (13, 0) -> (31.75, 0)
  arc A9 (31.75, -0.1016) -> (31.75, 0.1016) centre (31.75, 0) ccw
  arc A10 (13, 0.1016) -> (13, -0.1016) centre (13, 0) ccw
  arc A11 (31.75, 0) -> (36.83, 5.08) centre (31.75, 5.08) ccw
  arc A12 (31.75, 0.1016) -> (31.75, -0.1016) centre (31.75, 0) ccw
  arc A13 (36.9316, 5.08) -> (36.7284, 5.08) centre (36.83, 5.08) ccw
  line L3 (36.83, 5.08) -> (36.83, 6.5)
  arc A14 (36.9316, 6.5) -> (36.7284, 6.5) centre (36.83, 6.5) ccw
  arc A15 (36.7284, 5.08) -> (36.9316, 5.08) centre (36.83, 5.08) ccw
  line L4 (36.83, 13) -> (36.83, 32.766)
  arc A16 (36.9316, 32.766) -> (36.7284, 32.766) centre (36.83, 32.766) ccw
  arc A17 (36.7284, 13) -> (36.9316, 13) centre (36.83, 13) ccw
  arc A18 (36.83, 32.766) -> (32.766, 36.83) centre (32.766, 32.766) ccw
  arc A19 (36.7284, 32.766) -> (36.9316, 32.766) centre (36.83, 32.766) ccw
  arc A20 (32.766, 36.9316) -> (32.766, 36.7284) centre (32.766, 36.83) ccw
  line L5 (32.766, 36.83) -> (13, 36.83)
  arc A21 (13, 36.9316) -> (13, 36.7284) centre (13, 36.83) ccw
  arc A22 (32.766, 36.7284) -> (32.766, 36.9316) centre (32.766, 36.83) ccw
  line L6 (6.5, 36.83) -> (5.08, 36.83)
  arc A23 (5.08, 36.9316) -> (5.08, 36.7284) centre (5.08, 36.83) ccw
  arc A24 (6.5, 36.7284) -> (6.5, 36.9316) centre (6.5, 36.83) ccw
  arc A25 (5.08, 36.83) -> (0, 31.75) centre (5.08, 31.75) ccw
  arc A26 (5.08, 36.7284) -> (5.08, 36.9316) centre (5.08, 36.83) ccw
  arc A27 (-0.1016, 31.75) -> (0.1016, 31.75) centre (0, 31.75) ccw
  arc A28 (0, 6.5) -> (0, 13) centre (-1.4083, 9.75) ccw
  arc A29 (-0.0404, 6.5932) -> (0.0404, 6.4068) centre (0, 6.5) ccw
  arc A30 (0.0404, 13.0932) -> (-0.0404, 12.9068) centre (0, 13) ccw
  arc A31 (13, 0) -> (6.5, 0) centre (9.75, -1.4083) ccw
  arc A32 (12.9068, -0.0404) -> (13.0932, 0.0404) centre (13, 0) ccw
  arc A33 (6.4068, 0.0404) -> (6.5932, -0.0404) centre (6.5, 0) ccw
  arc A34 (36.83, 13) -> (36.83, 6.5) centre (38.2383, 9.75) ccw
  arc A35 (36.8704, 12.9068) -> (36.7896, 13.0932) centre (36.83, 13) ccw
  arc A36 (36.7896, 6.4068) -> (36.8704, 6.5932) centre (36.83, 6.5) ccw
  arc A37 (6.5, 36.83) -> (13, 36.83) centre (9.75, 38.2383) ccw
  arc A38 (6.5932, 36.8704) -> (6.4068, 36.7896) centre (6.5, 36.83) ccw
  arc A39 (13.0932, 36.7896) -> (12.9068, 36.8704) centre (13, 36.83) ccw
  circle A40 centre (6.604, 32.258) radius 0.5
  circle A41 centre (14.224, 31.242) radius 0.5
  circle A42 centre (14.224, 33.274) radius 0.5
  circle A43 centre (3.302, 34.036) radius 1.016
  circle A44 centre (34.036, 3.302) radius 1.016
  circle A45 centre (34.29, 34.29) radius 1.016
  line L7 (0, 31.75) -> (0, 13)
  circle A46 centre (2.794, 3.048) radius 1.016
  constraints: 100 point on circle, 47 centre point, 16 end point, 6 point on line
sketch "21" plane through (0, 0, 0) normal (0, 0, 1) x (1, 0, 0)
  arc A0 (25.9121, 5.3101) -> (25.948, 5.2742) centre (25.93, 5.2922) ccw
  line L0 (25.93, 5.8434) -> (26.4813, 5.2922)
  arc A1 (26.4633, 5.2742) -> (26.4993, 5.3101) centre (26.4813, 5.2922) ccw
  arc A2 (6.604, 29.7497) -> (6.604, 29.6862) centre (6.604, 29.718) ccw
  arc A3 (25.948, 5.8614) -> (25.9121, 5.8255) centre (25.93, 5.8434) ccw
  line L1 (5.2755, 25.9467) -> (5.8267, 26.498)
  arc A4 (5.8447, 26.48) -> (5.8087, 26.516) centre (5.8267, 26.498) ccw
  arc A5 (5.2575, 25.9647) -> (5.2934, 25.9288) centre (5.2755, 25.9467) ccw
  arc A6 (13.7, 3.716) -> (13.7, 23.716) centre (13.7, 13.716) ccw
  arc A7 (13.7, 23.716) -> (13.7, 3.716) centre (13.7, 13.716) ccw
  arc A8 (26.1825, 4.6459) -> (26.1825, 6.442) centre (26.1825, 5.544) ccw
  arc A9 (26.1825, 6.442) -> (26.1825, 4.6459) centre (26.1825, 5.544) ccw
  arc A10 (5.528, 25.3005) -> (5.528, 27.0966) centre (5.528, 26.1986) ccw
  arc A11 (5.528, 27.0966) -> (5.528, 25.3005) centre (5.528, 26.1986) ccw
  line L2 (27.5213, 15.7387) -> (14.7227, 28.5373)
  arc A12 (14.7451, 28.5598) -> (14.7002, 28.5149) centre (14.7227, 28.5373) ccw
  arc A13 (27.4989, 15.7162) -> (27.5438, 15.7611) centre (27.5213, 15.7387) ccw
  line L3 (14.7227, 28.5373) -> (23.2433, 37.058)
  arc A14 (23.2658, 37.0355) -> (23.2209, 37.0804) centre (23.2433, 37.058) ccw
  arc A15 (14.7002, 28.5598) -> (14.7451, 28.5149) centre (14.7227, 28.5373) ccw
  line L4 (23.2433, 37.058) -> (36.042, 24.2593)
  arc A16 (36.0195, 24.2369) -> (36.0644, 24.2818) centre (36.042, 24.2593) ccw
  arc A17 (23.2658, 37.0804) -> (23.2209, 37.0355) centre (23.2433, 37.058) ccw
  line L5 (36.042, 24.2593) -> (27.5213, 15.7387)
  arc A18 (27.4989, 15.7611) -> (27.5438, 15.7162) centre (27.5213, 15.7387) ccw
  arc A19 (36.0644, 24.2369) -> (36.0195, 24.2818) centre (36.042, 24.2593) ccw
  line L6 (16.4611, 29.2569) -> (16.4611, 29.6045)
  arc A20 (16.4802, 29.6045) -> (16.4421, 29.6045) centre (16.4611, 29.6045) ccw
  arc A21 (16.4421, 29.2569) -> (16.4802, 29.2569) centre (16.4611, 29.2569) ccw
  line L7 (16.4611, 29.6045) -> (16.9824, 29.0832)
  arc A22 (16.9689, 29.0697) -> (16.9959, 29.0966) centre (16.9824, 29.0832) ccw
  arc A23 (16.4746, 29.6179) -> (16.4476, 29.591) centre (16.4611, 29.6045) ccw
  line L8 (16.8086, 28.9094) -> (17.1562, 29.2569)
  arc A24 (17.1697, 29.2435) -> (17.1427, 29.2704) centre (17.1562, 29.2569) ccw
  arc A25 (16.7952, 28.9229) -> (16.8221, 28.8959) centre (16.8087, 28.9094) ccw
  line L9 (27.1031, 18.615) -> (27.1031, 18.9625)
  arc A26 (27.1221, 18.9625) -> (27.084, 18.9625) centre (27.1031, 18.9625) ccw
  arc A27 (27.084, 18.615) -> (27.1221, 18.615) centre (27.1031, 18.615) ccw
  line L10 (27.1031, 18.9625) -> (27.6244, 18.4412)
  arc A28 (27.6109, 18.4277) -> (27.6378, 18.4547) centre (27.6244, 18.4412) ccw
  arc A29 (27.1166, 18.976) -> (27.0896, 18.949) centre (27.1031, 18.9625) ccw
  arc A30 (33.158, 23.9939) -> (33.1961, 23.9939) centre (33.177, 23.9939) ccw
  line L11 (27.4506, 18.2675) -> (27.7981, 18.615)
  arc A31 (27.8116, 18.6015) -> (27.7847, 18.6284) centre (27.7981, 18.615) ccw
  arc A32 (27.4371, 18.2809) -> (27.4641, 18.254) centre (27.4506, 18.2674) ccw
  line L12 (27.5454, 19.231) -> (27.5454, 19.4048)
  arc A33 (27.5644, 19.4048) -> (27.5263, 19.4048) centre (27.5454, 19.4048) ccw
  arc A34 (27.5263, 19.231) -> (27.5644, 19.231) centre (27.5454, 19.231) ccw
  line L13 (27.5454, 19.4048) -> (27.7192, 19.5786)
  arc A35 (27.7326, 19.5651) -> (27.7057, 19.5921) centre (27.7192, 19.5786) ccw
  arc A36 (27.5319, 19.4183) -> (27.5589, 19.3913) centre (27.5454, 19.4048) ccw
  line L14 (27.7192, 19.5786) -> (27.8931, 19.5786)
  arc A37 (27.8931, 19.5596) -> (27.8931, 19.5977) centre (27.8931, 19.5786) ccw
  arc A38 (27.7192, 19.5976) -> (27.7192, 19.5595) centre (27.7192, 19.5786) ccw
  line L15 (27.8931, 19.5786) -> (27.9799, 19.4917)
  arc A39 (27.9664, 19.4782) -> (27.9934, 19.5052) centre (27.9799, 19.4917) ccw
  arc A40 (27.9065, 19.5921) -> (27.8796, 19.5652) centre (27.8931, 19.5786) ccw
  line L16 (27.9799, 19.4917) -> (27.9798, 19.3179)
  arc A41 (27.9608, 19.3179) -> (27.9989, 19.3179) centre (27.9798, 19.3179) ccw
  arc A42 (27.999, 19.4917) -> (27.9609, 19.4917) centre (27.9799, 19.4917) ccw
  line L17 (27.9798, 19.3179) -> (27.8929, 19.231)
  arc A43 (27.8795, 19.2445) -> (27.9064, 19.2176) centre (27.8929, 19.2311) ccw
  arc A44 (27.9933, 19.3045) -> (27.9663, 19.3314) centre (27.9798, 19.3179) ccw
  line L18 (27.9798, 19.3179) -> (28.1536, 19.3179)
  arc A45 (28.1536, 19.2989) -> (28.1536, 19.337) centre (28.1536, 19.3179) ccw
  arc A46 (27.9798, 19.337) -> (27.9798, 19.2989) centre (27.9798, 19.3179) ccw
  line L19 (28.1536, 19.3179) -> (28.2404, 19.231)
  arc A47 (28.227, 19.2176) -> (28.2539, 19.2445) centre (28.2405, 19.2311) ccw
  arc A48 (28.167, 19.3314) -> (28.1401, 19.3045) centre (28.1536, 19.3179) ccw
  line L20 (28.2404, 19.231) -> (28.2404, 19.0573)
  arc A49 (28.2214, 19.0573) -> (28.2595, 19.0573) centre (28.2404, 19.0573) ccw
  arc A50 (28.2595, 19.231) -> (28.2214, 19.231) centre (28.2404, 19.231) ccw
  line L21 (28.2404, 19.0573) -> (28.0667, 18.8835)
  arc A51 (28.0532, 18.897) -> (28.0802, 18.8701) centre (28.0667, 18.8835) ccw
  arc A52 (28.2539, 19.0438) -> (28.227, 19.0708) centre (28.2405, 19.0573) ccw
  line L22 (28.0667, 18.8835) -> (27.8929, 18.8835)
  arc A53 (27.8929, 18.9026) -> (27.8929, 18.8645) centre (27.8929, 18.8835) ccw
  arc A54 (28.0667, 18.8645) -> (28.0667, 18.9026) centre (28.0667, 18.8835) ccw
  line L23 (32.9954, 23.8122) -> (32.6478, 23.4647)
  arc A55 (32.6344, 23.4781) -> (32.6613, 23.4512) centre (32.6478, 23.4647) ccw
  arc A56 (33.0088, 23.7987) -> (32.9819, 23.8257) centre (32.9954, 23.8122) ccw
  line L24 (32.6478, 23.4647) -> (32.6478, 24.1597)
  arc A57 (32.6669, 24.1597) -> (32.6288, 24.1597) centre (32.6478, 24.1597) ccw
  arc A58 (32.6288, 23.4647) -> (32.6669, 23.4647) centre (32.6478, 23.4647) ccw
  line L25 (32.6478, 24.1597) -> (32.561, 24.2466)
  arc A59 (32.5744, 24.2601) -> (32.5475, 24.2331) centre (32.561, 24.2466) ccw
  arc A60 (14.224, 29.6862) -> (14.224, 29.7497) centre (14.224, 29.718) ccw
  line L26 (6.604, 29.718) -> (14.224, 29.718)
  arc A61 (23.5995, 8.0591) -> (23.5995, 15.1302) centre (20.064, 11.5947) ccw
  arc A62 (23.577, 8.0816) -> (23.6219, 8.0367) centre (23.5995, 8.0591) ccw
  arc A63 (23.622, 15.1527) -> (23.577, 15.1078) centre (23.5995, 15.1302) ccw
  line L27 (23.5995, 15.1302) -> (13.7566, 24.9731)
  arc A64 (13.779, 24.9956) -> (13.7341, 24.9507) centre (13.7566, 24.9731) ccw
  arc A65 (23.577, 15.1078) -> (23.622, 15.1527) centre (23.5995, 15.1302) ccw
  arc A66 (13.7566, 24.9731) -> (12.3423, 24.9731) centre (13.0495, 24.266) ccw
  arc A67 (13.7341, 24.9507) -> (13.779, 24.9956) centre (13.7566, 24.9731) ccw
  arc A68 (12.3199, 24.9956) -> (12.3648, 24.9507) centre (12.3424, 24.9731) ccw
  arc A69 (12.3423, 24.9731) -> (12.3423, 23.5589) centre (13.0494, 24.266) ccw
  arc A70 (12.3648, 24.9507) -> (12.3199, 24.9956) centre (12.3424, 24.9731) ccw
  arc A71 (12.3199, 23.5365) -> (12.3648, 23.5814) centre (12.3424, 23.5589) ccw
  line L28 (12.3423, 23.5589) -> (11.5787, 24.3226)
  arc A72 (11.6011, 24.3451) -> (11.5562, 24.3002) centre (11.5787, 24.3226) ccw
  arc A73 (12.3199, 23.5365) -> (12.3648, 23.5814) centre (12.3424, 23.5589) ccw
  line L29 (11.5787, 24.3226) -> (3.0934, 15.8373)
  arc A74 (3.0709, 15.8598) -> (3.1158, 15.8149) centre (3.0934, 15.8373) ccw
  arc A75 (11.6011, 24.3002) -> (11.5562, 24.3451) centre (11.5787, 24.3226) ccw
  line L30 (3.0934, 15.8373) -> (3.8571, 15.0737)
  arc A76 (3.8346, 15.0512) -> (3.8795, 15.0961) centre (3.8571, 15.0736) ccw
  arc A77 (3.1158, 15.8598) -> (3.0709, 15.8149) centre (3.0934, 15.8373) ccw
  arc A78 (3.8571, 15.0737) -> (2.4429, 15.0737) centre (3.15, 14.3666) ccw
  arc A79 (3.8346, 15.0512) -> (3.8795, 15.0961) centre (3.8571, 15.0736) ccw
  arc A80 (2.4204, 15.0961) -> (2.4653, 15.0512) centre (2.4429, 15.0736) ccw
  arc A81 (2.4429, 15.0737) -> (2.4429, 13.6594) centre (3.15, 14.3665) ccw
  arc A82 (32.6344, 24.1463) -> (32.6613, 24.1732) centre (32.6478, 24.1597) ccw
  line L31 (32.561, 24.2466) -> (32.3872, 24.2466)
  arc A83 (32.3872, 24.2657) -> (32.3872, 24.2276) centre (32.3872, 24.2466) ccw
  arc A84 (32.561, 24.2276) -> (32.561, 24.2657) centre (32.561, 24.2466) ccw
  line L32 (32.3872, 24.2466) -> (32.2134, 24.0728)
  arc A85 (32.2, 24.0863) -> (32.2269, 24.0594) centre (32.2134, 24.0728) ccw
  arc A86 (32.4007, 24.2331) -> (32.3737, 24.2601) centre (32.3872, 24.2466) ccw
  line L33 (32.2134, 24.0728) -> (32.2134, 23.8991)
  arc A87 (32.1944, 23.8991) -> (32.2325, 23.8991) centre (32.2134, 23.8991) ccw
  arc A88 (32.2325, 24.0728) -> (32.1944, 24.0728) centre (32.2134, 24.0728) ccw
  line L34 (33.5246, 24.3414) -> (33.177, 23.9939)
  arc A89 (33.1636, 24.0074) -> (33.1905, 23.9804) centre (33.1771, 23.9939) ccw
  arc A90 (33.5381, 24.3279) -> (33.5111, 24.3549) centre (33.5246, 24.3414) ccw
  line L35 (33.177, 23.9939) -> (33.177, 24.689)
  arc A91 (33.1961, 24.689) -> (33.158, 24.689) centre (33.177, 24.689) ccw
  arc A92 (2.4653, 15.0512) -> (2.4204, 15.0961) centre (2.4429, 15.0736) ccw
  line L36 (33.177, 24.689) -> (33.0902, 24.7758)
  arc A93 (33.1036, 24.7893) -> (33.0767, 24.7624) centre (33.0902, 24.7758) ccw
  arc A94 (33.1636, 24.6755) -> (33.1905, 24.7024) centre (33.1771, 24.6889) ccw
  line L37 (33.0902, 24.7758) -> (32.9164, 24.7758)
  arc A95 (32.9164, 24.7949) -> (32.9164, 24.7568) centre (32.9164, 24.7758) ccw
  arc A96 (33.0902, 24.7568) -> (33.0902, 24.7949) centre (33.0902, 24.7758) ccw
  line L38 (32.9164, 24.7758) -> (32.7426, 24.6021)
  arc A97 (32.7292, 24.6155) -> (32.7561, 24.5886) centre (32.7426, 24.6021) ccw
  arc A98 (32.9299, 24.7624) -> (32.9029, 24.7893) centre (32.9164, 24.7758) ccw
  line L39 (32.7426, 24.6021) -> (32.7426, 24.4283)
  arc A99 (32.7236, 24.4283) -> (32.7617, 24.4283) centre (32.7426, 24.4283) ccw
  arc A100 (32.7617, 24.6021) -> (32.7236, 24.6021) centre (32.7426, 24.6021) ccw
  line L40 (25.1424, 30.9701) -> (25.1424, 31.1439)
  arc A101 (25.1614, 31.1439) -> (25.1233, 31.1439) centre (25.1424, 31.1439) ccw
  arc A102 (25.1233, 30.9701) -> (25.1614, 30.9702) centre (25.1424, 30.9702) ccw
  line L41 (25.1424, 31.1439) -> (25.3161, 31.3177)
  arc A103 (25.3296, 31.3042) -> (25.3026, 31.3312) centre (25.3161, 31.3177) ccw
  arc A104 (25.1289, 31.1574) -> (25.1558, 31.1304) centre (25.1423, 31.1439) ccw
  line L42 (25.3161, 31.3177) -> (25.49, 31.3177)
  arc A105 (25.49, 31.2987) -> (25.49, 31.3368) centre (25.49, 31.3177) ccw
  arc A106 (25.3161, 31.3367) -> (25.3161, 31.2986) centre (25.3161, 31.3177) ccw
  line L43 (25.49, 31.3177) -> (25.5769, 31.2308)
  arc A107 (25.5634, 31.2173) -> (25.5903, 31.2443) centre (25.5769, 31.2308) ccw
  arc A108 (25.5035, 31.3312) -> (25.4765, 31.3042) centre (25.49, 31.3177) ccw
  line L44 (25.5769, 31.2308) -> (25.5768, 31.057)
  arc A109 (25.5577, 31.057) -> (25.5958, 31.057) centre (25.5768, 31.057) ccw
  arc A110 (25.5959, 31.2308) -> (25.5578, 31.2308) centre (25.5769, 31.2308) ccw
  line L45 (25.5768, 31.057) -> (25.4899, 30.9701)
  arc A111 (25.4764, 30.9836) -> (25.5033, 30.9567) centre (25.4899, 30.9701) ccw
  arc A112 (25.5902, 31.0436) -> (25.5633, 31.0705) centre (25.5768, 31.057) ccw
  line L46 (25.5768, 31.057) -> (25.7505, 31.057)
  arc A113 (25.7505, 31.038) -> (25.7505, 31.0761) centre (25.7505, 31.057) ccw
  arc A114 (25.5768, 31.0761) -> (25.5768, 31.038) centre (25.5768, 31.057) ccw
  line L47 (25.7505, 31.057) -> (25.8374, 30.9701)
  arc A115 (25.824, 30.9567) -> (25.8509, 30.9836) centre (25.8374, 30.9702) ccw
  arc A116 (25.764, 31.0705) -> (25.737, 31.0436) centre (25.7505, 31.057) ccw
  line L48 (25.8374, 30.9701) -> (25.8374, 30.7964)
  arc A117 (25.8183, 30.7964) -> (25.8564, 30.7964) centre (25.8374, 30.7964) ccw
  arc A118 (25.8564, 30.9701) -> (25.8183, 30.9702) centre (25.8374, 30.9701) ccw
  line L49 (25.8374, 30.7964) -> (25.6636, 30.6226)
  arc A119 (25.6502, 30.6361) -> (25.6771, 30.6092) centre (25.6636, 30.6226) ccw
  arc A120 (25.8509, 30.7829) -> (25.8239, 30.8099) centre (25.8374, 30.7964) ccw
  line L50 (25.6636, 30.6226) -> (25.4899, 30.6226)
  arc A121 (25.4899, 30.6417) -> (25.4899, 30.6036) centre (25.4899, 30.6226) ccw
  arc A122 (25.6636, 30.6036) -> (25.6636, 30.6417) centre (25.6636, 30.6226) ccw
  line L51 (26.0191, 31.1518) -> (25.6716, 31.4994)
  arc A123 (25.685, 31.5128) -> (25.6581, 31.4859) centre (25.6716, 31.4994) ccw
  arc A124 (26.0569, 30.9973) -> (26.1252, 31.1624) centre (26.091, 31.0799) ccw
  line L52 (25.6716, 31.4994) -> (25.6716, 31.6731)
  arc A125 (25.6906, 31.6731) -> (25.6525, 31.6731) centre (25.6716, 31.6731) ccw
  arc A126 (25.6525, 31.4994) -> (25.6906, 31.4994) centre (25.6716, 31.4994) ccw
  line L53 (25.6716, 31.6731) -> (25.8453, 31.8469)
  arc A127 (25.8588, 31.8334) -> (25.8319, 31.8604) centre (25.8453, 31.8469) ccw
  arc A128 (25.6581, 31.6866) -> (25.685, 31.6596) centre (25.6716, 31.6731) ccw
  line L54 (25.8453, 31.8469) -> (25.3241, 31.8469)
  arc A129 (25.3375, 31.8334) -> (25.3241, 31.8659) centre (25.3241, 31.8469) ccw
  arc A130 (25.8453, 31.8659) -> (25.8453, 31.8278) centre (25.8453, 31.8469) ccw
  line L55 (25.3241, 31.8469) -> (25.7781, 31.6588)
  arc A131 (26.3532, 31.4859) -> (26.3801, 31.5128) centre (26.3666, 31.4994) ccw
  arc A132 (25.3375, 31.8604) -> (25.3106, 31.8334) centre (25.3241, 31.8469) ccw
  line L56 (25.7781, 31.6588) -> (26.3666, 31.3256)
  arc A133 (26.3476, 31.3256) -> (26.3857, 31.3256) centre (26.3666, 31.3256) ccw
  arc A134 (25.6994, 31.7142) -> (25.6613, 31.7142) centre (25.6803, 31.7142) ccw
  line L57 (26.3666, 31.3256) -> (26.1929, 31.1518)
  arc A135 (26.1794, 31.1653) -> (26.2063, 31.1384) centre (26.1929, 31.1518) ccw
  arc A136 (26.3801, 31.3121) -> (26.3531, 31.3391) centre (26.3666, 31.3256) ccw
  line L58 (26.1929, 31.1518) -> (26.0191, 31.1518)
  arc A137 (26.0056, 31.1653) -> (26.0191, 31.1328) centre (26.0191, 31.1518) ccw
  arc A138 (26.1929, 31.1328) -> (26.1929, 31.1709) centre (26.1929, 31.1518) ccw
  line L59 (26.0191, 31.1518) -> (25.3241, 31.8469)
  arc A139 (25.3431, 31.8469) -> (25.305, 31.8469) centre (25.3241, 31.8469) ccw
  arc A140 (26, 31.1518) -> (26.0381, 31.1518) centre (26.0191, 31.1518) ccw
  arc A141 (2.4204, 13.637) -> (2.4653, 13.6819) centre (2.4429, 13.6594) ccw
  line L60 (2.4429, 13.6594) -> (12.2858, 3.8165)
  arc A142 (12.2633, 3.794) -> (12.3082, 3.839) centre (12.2858, 3.8165) ccw
  arc A143 (2.4653, 13.6819) -> (2.4204, 13.637) centre (2.4429, 13.6594) ccw
  arc A144 (12.2858, 3.8165) -> (19.3569, 3.8165) centre (15.8213, 7.352) ccw
  arc A145 (12.3082, 3.839) -> (12.2633, 3.794) centre (12.2858, 3.8165) ccw
  arc A146 (19.3793, 3.794) -> (19.3344, 3.839) centre (19.3569, 3.8165) ccw
  line L61 (19.3569, 3.8165) -> (23.5995, 8.0591)
  arc A147 (23.6219, 8.0367) -> (23.577, 8.0816) centre (23.5995, 8.0591) ccw
  arc A148 (19.3344, 3.839) -> (19.3793, 3.794) centre (19.3569, 3.8165) ccw
  line L62 (25.93, 5.2922) -> (26.4813, 5.8434)
  arc A149 (26.4993, 5.8255) -> (26.4633, 5.8614) centre (26.4813, 5.8434) ccw
  constraints: 362 point on circle, 150 centre point, 126 end point, 49 point on line, 4 midpoint